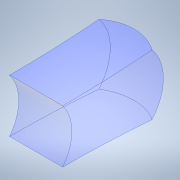
# Autodesk Inventor part: shank_2
Saved by Autodesk Inventor 2020.2 (Build 242310000, 310)
## iProperties
Created: 2021-01-30
Part Number: shank_2
Material: Generic
Document SubType Name: Modeling
Designer: DELL
Density: 1 g/cm^3
Appearance: Clear - Blue
Author: DELL
Autodesk Inventor part; units mm, degrees
ref_plane "Work Plane2" through (0, -32.5, -80) normal (0, 0, -1) x (0, 1, 0)
ref_plane "Work Plane1" through (0, 0, 27.5) normal (0, 0, 1) x (1, 0, 0)
ref_plane "Work Plane3" through (0, 0, -200) normal (0, 0, -1) x (-1, 0, 0)
sketch "Sketch11" plane through (0, 0, 0) normal (1, 0, 0) x (0, 1, 0)
  line L0 (-309.4604, 0) -> (1517.2621, 0) construction
  line L1 (0, -249.7) -> (0, 98.2) projected
  circle A0 centre (0, 0) radius 32.5
  circle A1 centre (0, 0) radius 48.5
  line L2 (-30, -38.1084) -> (-30, -151.9615)
  line L3 (-30, -151.9615) -> (30, -151.9615)
  line L4 (30, -151.9615) -> (30, -38.1084)
  arc A2 (-30, -151.9615) -> (30, -151.9615) centre (0, -100) ccw
  arc A3 (30, -151.9615) -> (50, -133.1662) centre (0, -100) ccw
  line L5 (0, -180) -> (50, -180)
  line L6 (50, -180) -> (50, -133.1662)
  arc A4 (30, -38.1084) -> (35, -148.734) centre (1256.3018, -38.1084) ccw
  point P0 (-30, -151.9615)
  point P1 (0, -160)
  point P2 (0, -151.9615)
  point P3 (0, -185.7103)
  point P4 (0, -160)
  point P5 (0, -48.5)
  dimension "d77" = 65
  dimension "d78" = 97
  dimension "d79" = 60
  dimension "d85" = 20
  dimension "d86" = 20
  dimension "d87" = 60
  dimension "d89" = 35
  dimension "d90" = 160
  constraints: 10 end point, 10 point on circle, 5 centre point, 3 coincident, 3 point on line, 2 perpendicular, 2 vertical, 1 horizontal, 1 tangent, 1 other
  measures "d77" diameter of A0
  measures "d78" diameter of A1
  measures "d79" distance between parallel lines of L4 L2
  measures "d85" distance edge to line of A2 L5
  measures "d86" distance from line of L4 L6.end
  measures "d87" radius of A2
  measures "d89" distance from line of A4.end L1
  measures "d90" distance of point (0, -160) A0.centre
extrude "Extrusion11" add sketch "Sketch11" along normal mid plane 60 contours L1 A1 L4 L3 | L4 A4 A3
revolve "Revolution1" add sketch "Sketch11" angle 180 mid plane about axis through (0, 0, -10) along (0, 0, 1) picked at (16.8404, -153.4348) contours L1 L3 A2
revolve "Revolution2" cut sketch "Sketch11" angle 360 about axis through (0, 0, -10) along (0, 0, 1) contours L1 A2 A3 L6 L5
mirror "Mirror1" about plane through (0, 0, 0) normal (0, 1, 0)
sketch "Sketch6" plane through (0, 0, 0) normal (1, 0, 0) x (0, 1, 0)
  circle A0 centre (0, 0) radius 32.5
  line L0 (-32.5, 0) -> (-32.5, -80)
  line L1 (-32.5, -80) -> (32.5, -80)
  line L2 (32.5, -80) -> (32.5, 0)
  line L3 (0, 0) -> (0, -80) construction
  line L4 (-32.5, -60) -> (32.5, -60)
  circle A1 centre (0, 0) radius 48.5
  point P0 (32.5, -36)
  point P1 (23.3184, -32.5)
  point P2 (0, -40)
  point P3 (-32.5, -36)
  dimension "d38" = 65
  dimension "d39" = 80
  dimension "d74" = 97
  dimension "d75" = 20
  dimension "d48" = 10
  dimension "d73" = 55
  dimension "d52" = 120
  constraints: 2 end point, 1 midpoint, 1 vertical
  measures "d52" distance from line of L0 L1.end
sketch "Sketch5" plane through (0, 0, -171) normal (0, 0, -1) x (-1, 0, 0)
  circle A0 centre (0, 0) radius 10
  point P0 (0, 0)
  dimension "d35" = 20
  constraints: 1 centre point, 1 coincident
  measures "d35" diameter of A0
body "Solid1"
body "Solid4"
body "Solid5"
